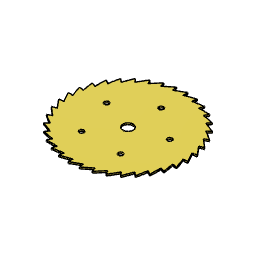
Braço robótico 3.0(serra disco) v2 (Autodesk Fusion 360 design; units mm, degrees)
Autodesk Fusion 360 part; units mm, degrees
sketch "Sketch1" plane through (0, 0, 0) normal (0, 1, 0) x (1, 0, 0)
  circle A0 centre (0, 0) radius 90 construction
  line L0 (-81.9196, 14.4446) -> (-88.6327, 15.6283)
  line L1 (-88.6327, 15.6283) -> (-83.1834, 0)
  line L2 (-90, 0) -> (-81.9196, -14.4446)
  line L3 (-83.1834, 0) -> (-90, 0)
  line L4 (-88.6327, -15.6283) -> (-78.1668, -28.4504)
  line L5 (-81.9196, -14.4446) -> (-88.6327, -15.6283)
  line L6 (-84.5723, -30.7818) -> (-72.0389, -41.5917)
  line L7 (-78.1668, -28.4504) -> (-84.5723, -30.7818)
  line L8 (-77.9423, -45) -> (-63.7222, -53.4693)
  line L9 (-72.0389, -41.5917) -> (-77.9423, -45)
  line L10 (-68.944, -57.8509) -> (-53.4693, -63.7222)
  line L11 (-63.7222, -53.4693) -> (-68.944, -57.8509)
  line L12 (-57.8509, -68.944) -> (-41.5917, -72.0389)
  line L13 (-53.4693, -63.7222) -> (-57.8509, -68.944)
  line L14 (-45, -77.9423) -> (-28.4504, -78.1668)
  line L15 (-41.5917, -72.0389) -> (-45, -77.9423)
  line L16 (-30.7818, -84.5723) -> (-14.4446, -81.9196)
  line L17 (-28.4504, -78.1668) -> (-30.7818, -84.5723)
  line L18 (-15.6283, -88.6327) -> (0, -83.1834)
  line L19 (-14.4446, -81.9196) -> (-15.6283, -88.6327)
  line L20 (0, -90) -> (14.4446, -81.9196)
  line L21 (0, -83.1834) -> (0, -90)
  line L22 (15.6283, -88.6327) -> (28.4504, -78.1668)
  line L23 (14.4446, -81.9196) -> (15.6283, -88.6327)
  line L24 (30.7818, -84.5723) -> (41.5917, -72.0389)
  line L25 (28.4504, -78.1668) -> (30.7818, -84.5723)
  line L26 (45, -77.9423) -> (53.4693, -63.7222)
  line L27 (41.5917, -72.0389) -> (45, -77.9423)
  line L28 (57.8509, -68.944) -> (63.7222, -53.4693)
  line L29 (53.4693, -63.7222) -> (57.8509, -68.944)
  line L30 (68.944, -57.8509) -> (72.0389, -41.5917)
  line L31 (63.7222, -53.4693) -> (68.944, -57.8509)
  line L32 (77.9423, -45) -> (78.1668, -28.4504)
  line L33 (72.0389, -41.5917) -> (77.9423, -45)
  line L34 (84.5723, -30.7818) -> (81.9196, -14.4446)
  line L35 (78.1668, -28.4504) -> (84.5723, -30.7818)
  line L36 (88.6327, -15.6283) -> (83.1834, 0)
  line L37 (81.9196, -14.4446) -> (88.6327, -15.6283)
  line L38 (90, 0) -> (81.9196, 14.4446)
  line L39 (83.1834, 0) -> (90, 0)
  line L40 (88.6327, 15.6283) -> (78.1668, 28.4504)
  line L41 (81.9196, 14.4446) -> (88.6327, 15.6283)
  line L42 (84.5723, 30.7818) -> (72.0389, 41.5917)
  line L43 (78.1668, 28.4504) -> (84.5723, 30.7818)
  line L44 (77.9423, 45) -> (63.7222, 53.4693)
  line L45 (72.0389, 41.5917) -> (77.9423, 45)
  line L46 (68.944, 57.8509) -> (53.4693, 63.7222)
  line L47 (63.7222, 53.4693) -> (68.944, 57.8509)
  line L48 (57.8509, 68.944) -> (41.5917, 72.0389)
  line L49 (53.4693, 63.7222) -> (57.8509, 68.944)
  line L50 (45, 77.9423) -> (28.4504, 78.1668)
  line L51 (41.5917, 72.0389) -> (45, 77.9423)
  line L52 (30.7818, 84.5723) -> (14.4446, 81.9196)
  line L53 (28.4504, 78.1668) -> (30.7818, 84.5723)
  line L54 (15.6283, 88.6327) -> (0, 83.1834)
  line L55 (14.4446, 81.9196) -> (15.6283, 88.6327)
  line L56 (0, 90) -> (-14.4446, 81.9196)
  line L57 (0, 83.1834) -> (0, 90)
  line L58 (-15.6283, 88.6327) -> (-28.4504, 78.1668)
  line L59 (-14.4446, 81.9196) -> (-15.6283, 88.6327)
  line L60 (-30.7818, 84.5723) -> (-41.5917, 72.0389)
  line L61 (-28.4504, 78.1668) -> (-30.7818, 84.5723)
  line L62 (-45, 77.9423) -> (-53.4693, 63.7222)
  line L63 (-41.5917, 72.0389) -> (-45, 77.9423)
  line L64 (-57.8509, 68.944) -> (-63.7222, 53.4693)
  line L65 (-53.4693, 63.7222) -> (-57.8509, 68.944)
  line L66 (-68.944, 57.8509) -> (-72.0389, 41.5917)
  line L67 (-63.7222, 53.4693) -> (-68.944, 57.8509)
  line L68 (-77.9423, 45) -> (-78.1668, 28.4504)
  line L69 (-72.0389, 41.5917) -> (-77.9423, 45)
  line L70 (-84.5723, 30.7818) -> (-81.9196, 14.4446)
  line L71 (-78.1668, 28.4504) -> (-84.5723, 30.7818)
  circle A1 centre (0, 0) radius 7.9405
  dimension "d1" = 180
  dimension "d5" = 15.881
  constraint coincident A0.centre A1.centre
  constraint coincident A0 L0.end
  measures "d1" diameter of A0
  measures "d5" diameter of A1
extrude "Extrude1" add sketch "Sketch1" along normal blind 2.32
sketch "Sketch2" plane through (0, 2.32, 0) normal (0, 1, 0) x (-1, 0, 0)
  circle A0 centre (0, 0) radius 7.9405
  line L0 (78.1668, -28.4504) -> (84.5723, -30.7818)
  line L1 (84.5723, -30.7818) -> (81.9196, -14.4446)
  line L2 (81.9196, -14.4446) -> (88.6327, -15.6283)
  line L3 (88.6327, -15.6283) -> (83.1834, 0)
  line L4 (83.1834, 0) -> (90, 0)
  line L5 (90, 0) -> (81.9196, 14.4446)
  line L6 (81.9196, 14.4446) -> (88.6327, 15.6283)
  line L7 (88.6327, 15.6283) -> (78.1668, 28.4504)
  line L8 (78.1668, 28.4504) -> (84.5723, 30.7818)
  line L9 (84.5723, 30.7818) -> (72.0389, 41.5917)
  line L10 (72.0389, 41.5917) -> (77.9423, 45)
  line L11 (77.9423, 45) -> (63.7222, 53.4693)
  line L12 (63.7222, 53.4693) -> (68.944, 57.8509)
  line L13 (68.944, 57.8509) -> (53.4693, 63.7222)
  line L14 (53.4693, 63.7222) -> (57.8509, 68.944)
  line L15 (57.8509, 68.944) -> (41.5917, 72.0389)
  line L16 (41.5917, 72.0389) -> (45, 77.9423)
  line L17 (45, 77.9423) -> (28.4504, 78.1668)
  line L18 (28.4504, 78.1668) -> (30.7818, 84.5723)
  line L19 (30.7818, 84.5723) -> (14.4446, 81.9196)
  line L20 (14.4446, 81.9196) -> (15.6283, 88.6327)
  line L21 (15.6283, 88.6327) -> (0, 83.1834)
  line L22 (0, 83.1834) -> (0, 90)
  line L23 (0, 90) -> (-14.4446, 81.9196)
  line L24 (-14.4446, 81.9196) -> (-15.6283, 88.6327)
  line L25 (-15.6283, 88.6327) -> (-28.4504, 78.1668)
  line L26 (-28.4504, 78.1668) -> (-30.7818, 84.5723)
  line L27 (-30.7818, 84.5723) -> (-41.5917, 72.0389)
  line L28 (-41.5917, 72.0389) -> (-45, 77.9423)
  line L29 (-45, 77.9423) -> (-53.4693, 63.7222)
  line L30 (-53.4693, 63.7222) -> (-57.8509, 68.944)
  line L31 (-57.8509, 68.944) -> (-63.7222, 53.4693)
  line L32 (-63.7222, 53.4693) -> (-68.944, 57.8509)
  line L33 (-68.944, 57.8509) -> (-72.0389, 41.5917)
  line L34 (-72.0389, 41.5917) -> (-77.9423, 45)
  line L35 (-77.9423, 45) -> (-78.1668, 28.4504)
  line L36 (-78.1668, 28.4504) -> (-84.5723, 30.7818)
  line L37 (-84.5723, 30.7818) -> (-81.9196, 14.4446)
  line L38 (-81.9196, 14.4446) -> (-88.6327, 15.6283)
  line L39 (-88.6327, 15.6283) -> (-83.1834, 0)
  line L40 (-83.1834, 0) -> (-90, 0)
  line L41 (-90, 0) -> (-81.9196, -14.4446)
  line L42 (-81.9196, -14.4446) -> (-88.6327, -15.6283)
  line L43 (-88.6327, -15.6283) -> (-78.1668, -28.4504)
  line L44 (-78.1668, -28.4504) -> (-84.5723, -30.7818)
  line L45 (-84.5723, -30.7818) -> (-72.0389, -41.5917)
  line L46 (-72.0389, -41.5917) -> (-77.9423, -45)
  line L47 (-77.9423, -45) -> (-63.7222, -53.4693)
  line L48 (-63.7222, -53.4693) -> (-68.944, -57.8509)
  line L49 (-68.944, -57.8509) -> (-53.4693, -63.7222)
  line L50 (-53.4693, -63.7222) -> (-57.8509, -68.944)
  line L51 (-57.8509, -68.944) -> (-41.5917, -72.0389)
  line L52 (-41.5917, -72.0389) -> (-45, -77.9423)
  line L53 (-45, -77.9423) -> (-28.4504, -78.1668)
  line L54 (-28.4504, -78.1668) -> (-30.7818, -84.5723)
  line L55 (-30.7818, -84.5723) -> (-14.4446, -81.9196)
  line L56 (-14.4446, -81.9196) -> (-15.6283, -88.6327)
  line L57 (-15.6283, -88.6327) -> (0, -83.1834)
  line L58 (0, -83.1834) -> (0, -90)
  line L59 (0, -90) -> (14.4446, -81.9196)
  line L60 (14.4446, -81.9196) -> (15.6283, -88.6327)
  line L61 (15.6283, -88.6327) -> (28.4504, -78.1668)
  line L62 (28.4504, -78.1668) -> (30.7818, -84.5723)
  line L63 (30.7818, -84.5723) -> (41.5917, -72.0389)
  line L64 (41.5917, -72.0389) -> (45, -77.9423)
  line L65 (45, -77.9423) -> (53.4693, -63.7222)
  line L66 (53.4693, -63.7222) -> (57.8509, -68.944)
  line L67 (57.8509, -68.944) -> (63.7222, -53.4693)
  line L68 (63.7222, -53.4693) -> (68.944, -57.8509)
  line L69 (68.944, -57.8509) -> (72.0389, -41.5917)
  line L70 (72.0389, -41.5917) -> (77.9423, -45)
  line L71 (77.9423, -45) -> (78.1668, -28.4504)
  circle A1 centre (0, -50) radius 3.5
  circle A2 centre (47.5528, -15.4508) radius 3.5
  circle A3 centre (29.3893, 40.4508) radius 3.5
  circle A4 centre (-29.3893, 40.4508) radius 3.5
  circle A5 centre (-47.5528, -15.4508) radius 3.5
  dimension "d8" = 7
  dimension "d10" = 360
  measures "d8" diameter of A1
extrude "Extrude2" cut sketch "Sketch2" against normal blind 30 contours A1 | A2 | A3 | A4 | A5
